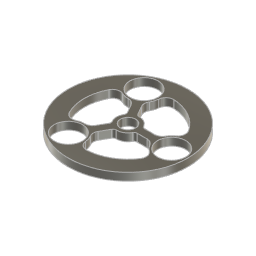
rgbRad v2 (Autodesk Fusion 360 design; units mm, degrees)
Autodesk Fusion 360 part; units mm, degrees
sketch "Skizze1" plane through (0, 0, 0) normal (0, 0, 1) x (1, 0, 0)
  circle A0 centre (0, 0) radius 78
  circle A1 centre (-28.5, 49.3634) radius 18.5
  circle A2 centre (57, 0) radius 18.5
  circle A3 centre (-28.5, -49.3634) radius 18.5
  line L0 (38.5, 0) -> (57, 0) construction
  arc A4 (47.8404, 30.9886) -> (2.9167, 56.9253) centre (0, 0) ccw
  arc A5 (-50.7571, 25.9367) -> (-50.7571, -25.9367) centre (0, 0) ccw
  arc A6 (2.9167, -56.9253) -> (47.8404, -30.9886) centre (0, 0) ccw
  line L1 (-19.2666, 23.3437) -> (-12.7215, 11.9321)
  line L2 (-4.16, 16.9974) -> (-10.6588, 28.3284)
  line L3 (-12.6985, -11.9728) -> (-19.2312, -23.349)
  line L4 (-10.6471, -28.3389) -> (-4.1337, -16.9965)
  line L5 (-7.5, -12.9904) -> (-18, -31.1769) construction
  line L6 (16.7914, -4.9152) -> (29.8791, -4.9572)
  line L7 (29.8309, 4.9862) -> (16.7051, 5.0283)
  arc A7 (-10.5378, 38.4842) -> (-7.5644, 47.7207) centre (-28.5, 49.3634) ccw
  arc A8 (-37.5452, 30.4113) -> (-28.1214, 28.3669) centre (-28.5, 49.3634) ccw
  arc A9 (-7.5644, -47.7207) -> (-10.5316, -38.4944) centre (-28.5, -49.3634) ccw
  arc A10 (-28.0956, -28.3673) -> (-37.5452, -30.4113) centre (-28.5, -49.3634) ccw
  arc A11 (38.606, -10.1322) -> (45.1095, -17.3094) centre (57, 0) ccw
  arc A12 (45.1095, 17.3094) -> (38.6169, 10.1519) centre (57, 0) ccw
  arc A13 (-12.7826, 7.8489) -> (-12.7637, -7.8797) centre (0, 0) ccw
  arc A14 (-0.525, -14.9908) -> (13.2462, -7.0383) centre (0, 0) ccw
  arc A15 (13.1984, 7.1276) -> (-0.5449, 14.9901) centre (0, 0) ccw
  arc A16 (13.1984, 7.1276) -> (16.7051, 5.0283) centre (16.718, 9.0283) ccw
  arc A17 (16.7914, -4.9152) -> (13.2462, -7.0383) centre (16.7786, -8.9151) ccw
  arc A18 (-0.525, -14.9908) -> (-4.1337, -16.9965) centre (-0.665, -18.9884) ccw
  arc A19 (-12.6985, -11.9728) -> (-12.7637, -7.8797) centre (-16.1673, -9.9809) ccw
  arc A20 (-12.7826, 7.8489) -> (-12.7215, 11.9321) centre (-16.1913, 9.942) ccw
  arc A21 (-4.16, 16.9974) -> (-0.5449, 14.9901) centre (-0.6902, 18.9875) ccw
  arc A22 (29.8309, 4.9862) -> (38.6169, 10.1519) centre (29.863, 14.9861) ccw
  arc A23 (38.606, -10.1322) -> (29.8791, -4.9572) centre (29.847, -14.9571) ccw
  arc A24 (-10.6471, -28.3389) -> (-10.5316, -38.4944) centre (-1.9752, -33.3187) ccw
  arc A25 (-28.0956, -28.3673) -> (-19.2312, -23.349) centre (-27.9031, -18.3692) ccw
  arc A26 (-19.2666, 23.3437) -> (-28.1214, 28.3669) centre (-27.9411, 18.3685) ccw
  arc A27 (-10.5378, 38.4842) -> (-10.6588, 28.3284) centre (-1.9843, 33.3036) ccw
  arc A28 (-37.5452, 30.4113) -> (-50.7571, 25.9367) centre (-41.8524, 21.3864) ccw
  arc A29 (2.9167, 56.9253) -> (-7.5644, 47.7207) centre (2.405, 46.9384) ccw
  arc A30 (45.1095, 17.3094) -> (47.8404, 30.9886) centre (39.4474, 25.552) ccw
  arc A31 (47.8404, -30.9886) -> (45.1095, -17.3094) centre (39.4474, -25.552) ccw
  arc A32 (-7.5644, -47.7207) -> (2.9167, -56.9253) centre (2.405, -46.9384) ccw
  arc A33 (-50.7571, -25.9367) -> (-37.5452, -30.4113) centre (-41.8524, -21.3864) ccw
  circle A34 centre (0, 0) radius 10
  dimension "d3" = 57
  dimension "d5" = 57
  dimension "d7" = 57
  dimension "d8" = 156
  dimension "d9" = 37
  dimension "d10" = 37
  dimension "d11" = 37
  dimension "d12" = 114
  dimension "d13" = 42
  dimension "d14" = 42
  dimension "d15" = 42
  dimension "d16" = 30
  dimension "d20" = 4
  dimension "d21" = 10
  dimension "d22" = 10
  dimension "d23" = 10
  dimension "d24" = 10
  dimension "d25" = 10
  dimension "d26" = 10
  dimension "d27" = 10
  dimension "d28" = 10
  dimension "d29" = 10
  dimension "d30" = 10
  dimension "d31" = 10
  dimension "d32" = 10
  dimension "d35" = 20
  constraint coincident A0.centre A4.centre
  constraint coincident A2.centre L0.end
  constraint concentric A0 A4
  constraint concentric A1 A7
  constraint concentric A3 A9
  constraint coincident A2 L0.start
  constraint concentric A4 A5
  constraint concentric A5 A6
  constraint concentric A5 A13
  constraint parallel L1 L2
  constraint parallel L3 L4
  constraint parallel L6 L7
  constraint concentric A7 A8
  constraint concentric A9 A10
  constraint concentric A11 A12
  constraint concentric A13 A14
  constraint concentric A14 A15
  constraint tangent A15 A16
  constraint tangent L7 A16
  constraint tangent A14 A17
  constraint tangent L6 A17
  constraint equal A16 A17
  constraint tangent A14 A18
  constraint tangent L4 A18
  constraint equal A16 A18
  constraint tangent A13 A19
  constraint tangent L3 A19
  constraint equal A16 A19
  constraint tangent A13 A20
  constraint tangent L1 A20
  constraint equal A16 A20
  constraint tangent A15 A21
  constraint tangent L2 A21
  constraint equal A16 A21
  constraint tangent A12 A22
  constraint tangent L7 A22
  constraint tangent A11 A23
  constraint tangent L6 A23
  constraint tangent A9 A24
  constraint tangent L4 A24
  constraint tangent A10 A25
  constraint tangent L3 A25
  constraint tangent A8 A26
  constraint tangent L1 A26
  constraint tangent A7 A27
  constraint tangent L2 A27
  constraint tangent A5 A28
  constraint tangent A8 A28
  constraint tangent A4 A29
  constraint tangent A7 A29
  constraint tangent A4 A30
  constraint tangent A12 A30
  constraint tangent A6 A31
  constraint tangent A11 A31
  constraint tangent A6 A32
  constraint tangent A9 A32
  constraint tangent A5 A33
  constraint tangent A10 A33
  constraint concentric A14 A34
  measures "d3" distance of A0.centre A2.centre
  measures "d5" distance of A0.centre A3.centre
  measures "d7" distance of A0.centre A1.centre
  measures "d8" diameter of A0
  measures "d9" diameter of A1
  measures "d10" diameter of A2
  measures "d11" diameter of A3
  measures "d12" diameter of A4
  measures "d13" diameter of A11
  measures "d14" diameter of A7
  measures "d15" diameter of A9
  measures "d16" diameter of A13
  measures "d20" radius of A16
  measures "d21" radius of A22
  measures "d22" radius of A23
  measures "d23" radius of A24
  measures "d24" radius of A25
  measures "d25" radius of A26
  measures "d26" radius of A27
  measures "d27" radius of A28
  measures "d28" radius of A29
  measures "d29" radius of A30
  measures "d30" radius of A31
  measures "d31" radius of A32
  measures "d32" radius of A33
  measures "d35" diameter of A34
extrude "Extrusion2" add sketch "Skizze1" along normal blind 10
equation "d8 = ( 57 * 2 ) * 1 mm + 37 mm + 5 mm"
equation "d12 = ( 57 * 2 ) * 1 mm"
equation "d13 = 37 mm + 5 mm"
equation "d14 = 37 mm + 5 mm"
equation "d15 = 37 mm + 5 mm"
